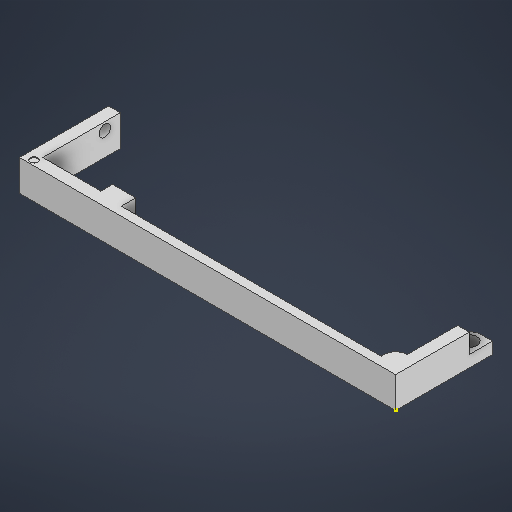
# Autodesk Inventor part: lewasciana
Saved by Autodesk Inventor 2026.2 (Build 302298010, 298A)
## iProperties
Created: 2026-04-27
Part Number: lewasciana
Material: Ogólny
Document SubType Name: Modeling
Designer: karol
Density: 1 g/cm^3
Appearance: Domyślna
Author: karol
Autodesk Inventor part; units mm, degrees
ref_plane "YZ Plane" through (0, 0, 0) normal (1, 0, 0) x (0, 1, 0)
ref_plane "XZ Plane" through (0, 0, 0) normal (0, 1, 0) x (-1, 0, 0)
ref_plane "XY Plane" through (0, 0, 0) normal (0, 0, 1) x (1, 0, 0)
sketch "Szkic1" plane through (0, 0, 0) normal (0, 1, 0) x (-1, 0, 0)
  line L0 (0, 0) -> (97, 0)
  line L1 (97, 0) -> (97, -3)
  line L2 (97, -3) -> (0, -3)
  line L3 (0, -3) -> (0, 0)
  dimension "d0" = 97
  dimension "d1" = 3
  constraints: 8 end point, 2 parallel, 1 horizontal, 1 perpendicular
  measures "d0" distance of L1.end L2.end
  measures "d1" distance of L0.end L1.end
extrude "Wyciągnięcie proste1" add sketch "Szkic1" along normal blind 8
sketch "Szkic2" plane through (0, 8, 0) normal (0, 1, 0) x (1, 0, 0)
  circle A0 centre (-94.6086, 1.3285) radius 1
  point P0 (0, 0)
  dimension "d4" = 2
  constraints: 1 centre point
  measures "d4" diameter of A0
extrude "Wyciągnięcie proste2" cut sketch "Szkic2" against normal blind 0.2
sketch "Szkic3" plane through (0, 0, -3) normal (0, 0, -1) x (-1, 0, 0)
  line L0 (0, 8) -> (97, 8) projected
  line L1 (0, 0) -> (3, 0)
  line L2 (3, 0) -> (3, 8)
  line L3 (3, 8) -> (0, 8)
  line L4 (0, 8) -> (0, 0)
  line L5 (0, 0) -> (97, 0) projected
  line L6 (97, 0) -> (94, 0)
  line L7 (94, 0) -> (94, 8)
  line L8 (94, 8) -> (97, 8)
  line L9 (97, 8) -> (97, 0)
  dimension "d7" = 3
  dimension "d8" = 3
  constraints: 16 end point, 4 parallel, 2 horizontal, 2 perpendicular, 2 point on line
  measures "d7" distance of L3.end L2.end
  measures "d8" distance of L7.end L8.end
extrude "Wyciągnięcie proste3" add sketch "Szkic3" along normal blind 19 contours L0 L2 L1 L4
extrude "Wyciągnięcie proste4" add sketch "Szkic3" along normal blind 20 contours L0 L9 L5 L7
sketch "Szkic4" plane through (-3, 0, -3) normal (-1, 0, 0) x (0, 0, 1)
  line L0 (-19, 0) -> (-19, 8) projected
  line L1 (0, 0) -> (-19, 0) projected
  line L2 (-19, 8) -> (-14, 8)
  line L3 (-14, 8) -> (-14, 0)
  line L4 (-14, 0) -> (-19, 0)
  line L5 (-19, 0) -> (-19, 8)
  point P0 (3, 0)
  dimension "d13" = 5
  constraints: 8 end point, 2 parallel, 1 horizontal, 1 perpendicular, 1 point on line
  measures "d13" distance of L3.end L4.end
extrude "Wyciągnięcie proste5" add sketch "Szkic4" along normal blind 3
sketch "Szkic5" plane through (0, 8, 0) normal (0, 1, 0) x (1, 0, 0)
  line L0 (-3, 3) -> (-3, 17) projected
  line L1 (-3, 3) -> (-6, 3)
  line L2 (-6, 3) -> (-6, 6)
  line L3 (-6, 6) -> (-3, 6)
  line L4 (-3, 6) -> (-3, 3)
  point P0 (0, 0)
  dimension "d16" = 3
  dimension "d17" = 3
  constraints: 8 end point, 2 parallel, 1 horizontal, 1 perpendicular
  measures "d16" distance of L2.end L3.end
  measures "d17" distance of L1.end L2.end
extrude "Wyciągnięcie proste6" add sketch "Szkic5" against normal blind 8
sketch "Szkic6" plane through (0, 8, 0) normal (0, 1, 0) x (1, 0, 0)
  line L0 (0, 0) -> (-6, 6)
  line L1 (-97, 0) -> (0, 0) projected
  line L2 (-6, 0) -> (0, 6)
  line L3 (0, 0) -> (0, 22) projected
  circle A0 centre (-3, 3) radius 2
  dimension "d20" = 4
  constraints: 4 end point, 2 point on line, 1 centre point, 1 midpoint
  measures "d20" diameter of A0
extrude "Wyciągnięcie proste7" cut sketch "Szkic6" against normal blind 8 contours A0 L2 L0 | L0 L2 A0 | L2 A0 L0 | L0 A0 L2
sketch "Szkic7" plane through (0, 8, 0) normal (0, 1, 0) x (1, 0, 0)
  circle A0 centre (-3, 3) radius 2 projected
  circle A1 centre (-3, 3) radius 2
  point P0 (0, 0)
  constraints: 1 centre point, 1 coincident
extrude "Wyciągnięcie proste8" add sketch "Szkic7" against normal blind 3
sketch "Szkic8" plane through (0, 8, 0) normal (0, 1, 0) x (1, 0, 0)
  line L0 (-6, 3) -> (-94, 3) projected
  line L1 (-79, 3) -> (-73, 3)
  line L2 (-73, 3) -> (-73, 6)
  line L3 (-73, 6) -> (-79, 6)
  line L4 (-79, 6) -> (-79, 3)
  line L5 (-3, 6) -> (-3, 17) projected
  point P0 (0, 0)
  dimension "d25" = 6
  dimension "d26" = 3
  dimension "d27" = 70
  constraints: 8 end point, 2 parallel, 1 horizontal, 1 perpendicular, 1 point on line
  measures "d25" distance of L3.end L2.end
  measures "d26" distance of L2.end L1.end
  measures "d27" distance from line of L5 L2.end
extrude "Wyciągnięcie proste9" add sketch "Szkic8" against normal blind 8
sketch "Szkic9" plane through (0, 8, 0) normal (0, 1, 0) x (1, 0, 0)
  line L0 (-73, 3) -> (-73, 6) projected
  line L1 (-73, 6) -> (-78.8804, 0)
  line L2 (-97, 0) -> (0, 0) projected
  line L3 (-79, 3) -> (-79, 6) projected
  line L4 (-79, 6) -> (-72.878, 0)
  circle A0 centre (-75.939, 3) radius 2
  dimension "d30" = 4
  constraints: 4 end point, 1 centre point, 1 midpoint, 1 perpendicular, 1 point on line
  measures "d30" diameter of A0
extrude "Wyciągnięcie proste10" cut sketch "Szkic9" against normal blind 8 contours A0 L4 L1 | L1 L4 A0 | L4 A0 L1 | L1 A0 L4
sketch "Szkic10" plane through (0, 8, 0) normal (0, 1, 0) x (1, 0, 0)
  circle A0 centre (-75.939, 3) radius 2 projected
  circle A1 centre (-75.939, 3) radius 2
  point P0 (0, 0)
  constraints: 1 centre point, 1 coincident
extrude "Wyciągnięcie proste11" add sketch "Szkic10" against normal blind 3
sketch "Szkic11" plane through (-6, 0, -3) normal (0, 0, -1) x (-1, 0, 0)
  line L0 (67, 8) -> (67, 0) projected
  line L1 (91, 0) -> (-6, 0) projected
  line L2 (67, 8) -> (54, 8)
  line L3 (54, 8) -> (54, 0)
  line L4 (54, 0) -> (67, 0)
  line L5 (67, 0) -> (67, 8)
  dimension "d35" = 13
  constraints: 8 end point, 2 parallel, 1 horizontal, 1 perpendicular, 1 point on line
  measures "d35" distance of L4.end L3.end
extrude "Wyciągnięcie proste12" cut sketch "Szkic11" against normal blind 0.5
sketch "Szkic13" plane through (-6, 0, -3) normal (0, 0, -1) x (-1, 0, 0)
  line L0 (54, 0) -> (54, 8) projected
  line L1 (0, 0) -> (0, 8) projected
  line L2 (54, 8) -> (0, 8)
  line L3 (0, 8) -> (0, 0)
  line L4 (0, 0) -> (54, 0)
  line L5 (54, 0) -> (54, 8)
  point P0 (-6, 0)
  constraints: 8 end point, 2 parallel, 1 horizontal, 1 perpendicular
extrude "Wyciągnięcie proste14" cut sketch "Szkic13" against normal blind 0.75
sketch "Szkic14" plane through (-6, 0, -2.5) normal (0, 0, -1) x (-1, 0, 0)
  line L0 (67, 0) -> (54, 0) projected
  line L1 (67, 8) -> (67, 0) projected
  line L2 (54, 0) -> (67, 0)
  line L3 (67, 0) -> (67, 8)
  line L4 (67, 8) -> (54, 8)
  line L5 (54, 8) -> (54, 0)
  point P0 (-6, 0)
  constraints: 8 end point, 2 parallel, 1 horizontal, 1 perpendicular
extrude "Wyciągnięcie proste15" cut sketch "Szkic14" against normal blind 0.25
sketch "Szkic15" plane through (-97, 0, 0) normal (-1, 0, 0) x (0, 0, 1)
  circle A0 centre (-19, 6) radius 1.5
  line L0 (-23, 0) -> (-23, 8) projected
  line L1 (0, 8) -> (-23, 8) projected
  point P0 (0, 0)
  dimension "d44" = 3
  dimension "d45" = 4
  dimension "d46" = 2
  constraints: 1 centre point
  measures "d44" diameter of A0
  measures "d45" distance from line of L0 A0.centre
  measures "d46" distance from line of L1 A0.centre
extrude "Wyciągnięcie proste16" cut sketch "Szkic15" against normal up to surface (3 mm away)
sketch "Szkic16" plane through (0, 0, 0) normal (0, -1, 0) x (1, 0, 0)
  line L0 (-3, -6) -> (-3, -17) projected
  line L1 (-6, -22) -> (-6, -17) projected
  line L2 (-3, -17) -> (-6, -17)
  line L3 (-6, -17) -> (-6, -22)
  line L4 (-6, -22) -> (-3, -22)
  line L5 (-3, -22) -> (-3, -17)
  point P0 (0, 0)
  constraints: 8 end point, 2 parallel, 1 horizontal, 1 perpendicular
extrude "Wyciągnięcie proste17" cut sketch "Szkic16" against normal blind 8
sketch "Szkic17" plane through (0, 0, 0) normal (0, -1, 0) x (1, 0, 0)
  line L0 (0, 0) -> (0, -22) projected
  line L1 (0, -22) -> (-3, -22)
  line L2 (-3, -22) -> (-3, -19)
  line L3 (-3, -19) -> (0, -19)
  line L4 (0, -19) -> (0, -22)
  line L5 (0, -19) -> (-6, -19)
  line L6 (-6, -19) -> (-6, -25)
  line L7 (-6, -25) -> (0, -25)
  line L8 (0, -25) -> (0, -19)
  dimension "d51" = 3
  dimension "d52" = 3
  dimension "d53" = 6
  dimension "d54" = 6
  constraints: 16 end point, 4 parallel, 2 horizontal, 2 perpendicular
  measures "d51" distance of L2.end L3.end
  measures "d52" distance of L1.end L2.end
  measures "d53" distance of L7.end L6.end
  measures "d54" distance of L6.end L5.end
extrude "Wyciągnięcie proste18" add sketch "Szkic17" against normal blind 3 contours L8 L7 L6 L5 L2 L1
sketch "Szkic18" plane through (0, 8, 0) normal (0, 1, 0) x (1, 0, 0)
  line L0 (0, 22) -> (-3, 22) projected
  line L1 (-3, 22) -> (-3, 19) projected
  line L2 (0, 22) -> (-3, 22)
  line L3 (-3, 22) -> (-3, 19)
  line L4 (-3, 19) -> (0, 19)
  line L5 (0, 19) -> (0, 22)
  point P0 (0, 0)
  constraints: 8 end point, 2 parallel, 1 horizontal, 1 perpendicular
extrude "Wyciągnięcie proste19" cut sketch "Szkic18" against normal blind 5
sketch "Szkic19" plane through (0, 0, 0) normal (0, -1, 0) x (1, 0, 0)
  point P0 (0, 0)
sketch "Szkic20" plane through (0, 0, 0) normal (0, -1, 0) x (1, 0, 0)
  circle A0 centre (-3, -22) radius 2
  line L0 (-6, -25) -> (0, -25) projected
  line L1 (-6, -19) -> (-6, -25) projected
  point P0 (0, 0)
  point P1 (-6, -22)
  dimension "d59" = 4
  dimension "d60" = 3
  dimension "d61" = 3
  constraints: 1 centre point, 1 midpoint
  measures "d59" diameter of A0
  measures "d60" distance from line of L0 A0.centre
  measures "d61" distance of point (-6, -22) A0.centre
extrude "Wyciągnięcie proste20" cut sketch "Szkic20" against normal blind 3
fillet "Fillet1" radius 3 2 edges at (-6, 1.5, -25) (-6, 1.5, -19)
fillet "Fillet2" radius 3 1 edges at (-6, 4, -6)
